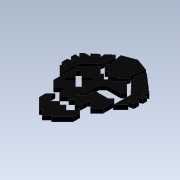
# Autodesk Inventor part: New Logo
Saved by Autodesk Inventor 2020 (Build 240168000, 168)
## iProperties
Created: 2021-10-28
Part Number: New Logo
Material: Generic
Document SubType Name: Modeling
Designer: Turing
Density: 1 g/cm^3
Appearance: Black Control Joints
Author: Turing
Autodesk Inventor part; units mm, degrees
ref_plane "YZ Plane" through (0, 0, 0) normal (1, 0, 0) x (0, 1, 0)
ref_plane "XZ Plane" through (0, 0, 0) normal (0, 1, 0) x (-1, 0, 0)
ref_plane "XY Plane" through (0, 0, 0) normal (0, 0, 1) x (1, 0, 0)
sketch "Sketch1" plane through (0, 0, 0) normal (0, 1, 0) x (-1, 0, 0)
  line L0 (0, 0) -> (-7.0711, -7.0711)
  line L1 (0, 0) -> (7.0711, -7.0711)
  line L2 (0, 0) -> (-1, 0)
  line L3 (7.0711, -7.0711) -> (17.6777, 3.5355)
  line L4 (-7.0711, -7.0711) -> (-17.6777, 3.5355)
  line L5 (0, 0) -> (0, 5)
  line L6 (0, 5) -> (7.0711, -2.0711)
  line L7 (7.0711, -2.0711) -> (17.6777, 8.5355)
  line L8 (0, 5) -> (-7.0711, -2.0711)
  line L9 (-7.0711, -2.0711) -> (-17.6777, 8.5355)
  line L10 (17.6777, 3.5355) -> (24.7487, -3.5355)
  line L11 (-17.6777, 3.5355) -> (-24.7487, -3.5355)
  line L12 (17.6777, 8.5355) -> (28.2843, -2.0711)
  line L13 (-17.6777, 8.5355) -> (-28.2843, -2.0711)
  line L14 (24.7487, -3.5355) -> (24.7487, -18.5355)
  line L15 (-24.7487, -3.5355) -> (-24.7487, -18.5355)
  line L16 (28.2843, -2.0711) -> (28.2843, -12.0711)
  line L17 (-28.2843, -2.0711) -> (-28.2843, -12.0711)
  line L18 (28.2843, -12.0711) -> (38.8909, -1.4645)
  line L19 (-28.2843, -12.0711) -> (-38.8909, -1.4645)
  line L20 (38.8909, -1.4645) -> (38.8909, 13.5355)
  line L21 (38.8909, 13.5355) -> (17.6777, 34.7487)
  line L22 (-38.8909, -1.4645) -> (-38.8909, 13.5355)
  line L23 (-38.8909, 13.5355) -> (-17.6777, 34.7487)
  line L24 (-17.6777, 34.7487) -> (17.6777, 34.7487)
  line L25 (24.7487, -18.5355) -> (28.2843, -22.0711)
  line L26 (28.2843, -22.0711) -> (42.4264, -7.9289)
  line L27 (-24.7487, -18.5355) -> (-28.2843, -22.0711)
  line L28 (-28.2843, -22.0711) -> (-42.4264, -7.9289)
  line L29 (17.6777, 34.7487) -> (14.1421, 38.2843)
  line L30 (14.1421, 38.2843) -> (10.6066, 34.7487)
  line L31 (0, 34.7487) -> (0, 45.7487)
  line L32 (10.6066, 34.7487) -> (0, 34.7487)
  line L33 (5.3033, 34.7487) -> (0, 34.7487)
  line L34 (0, 45.7487) -> (10.6066, 34.7487)
  line L35 (-17.6777, 34.7487) -> (-14.1421, 38.2843)
  line L36 (-14.1421, 38.2843) -> (-10.6066, 34.7487)
  line L37 (0, 45.7487) -> (-10.6066, 34.7487)
  line L38 (-42.4264, -7.9289) -> (-56.5685, -22.0711)
  line L39 (42.4264, -7.9289) -> (56.5685, -22.0711)
  line L40 (0, 0) -> (0, -18.5355)
  line L41 (0, -18.5355) -> (-10.6066, -29.1421)
  line L42 (-10.6066, -29.1421) -> (-10.6066, -44.1421)
  line L43 (-10.6066, -44.1421) -> (-14.1421, -47.6777)
  line L44 (-56.5685, -22.0711) -> (-56.5685, -47.6777)
  line L45 (-14.1421, -47.6777) -> (-56.5685, -47.6777)
  line L46 (-56.5685, -47.6777) -> (-49.4975, -54.7487)
  line L47 (-49.4975, -54.7487) -> (-42.4264, -47.6777)
  line L48 (-56.5685, -47.6777) -> (-52.6777, -47.6777)
  line L49 (-47.6777, -47.6777) -> (-42.4264, -47.6777)
  line L50 (-10.6066, -36.8853) -> (-5.6066, -36.8853)
  line L51 (-6.1919, -24.7274) -> (-2.6564, -28.263)
  line L52 (-5.6066, -36.8853) -> (-5.6066, -31.2132)
  line L53 (-5.6066, -31.2132) -> (-2.6564, -28.263)
  line L54 (0, -18.5355) -> (0, -25.6066)
  line L55 (0, -25.6066) -> (-2.6564, -28.263)
  line L56 (-5.6066, -36.8853) -> (-5.6066, -44.1422)
  line L57 (-5.6066, -44.1422) -> (-5.6066, -64.1422)
  line L58 (-5.6066, -64.1422) -> (-14.1421, -72.6777)
  line L59 (-14.1421, -72.6777) -> (-46.6651, -72.6777)
  line L60 (-46.6651, -72.6777) -> (-53.6117, -79.6243)
  line L61 (56.5685, -22.0711) -> (56.5685, -47.6777)
  line L62 (42.4264, -7.9289) -> (42.4264, -47.6786)
  line L63 (17.6777, 3.5355) -> (17.6777, -47.6786)
  line L64 (17.6777, -47.6786) -> (10.6066, -54.7497)
  line L65 (42.4264, -47.6786) -> (49.4975, -54.7497)
  line L66 (17.6777, -47.6786) -> (30.052, -60.053)
  line L67 (30.052, -60.053) -> (42.4264, -47.6786)
  line L68 (10.6066, -54.7497) -> (30.052, -74.1951)
  line L69 (30.052, -74.1951) -> (49.4975, -54.7497)
  line L70 (56.5685, -47.6777) -> (56.5685, -76.6674)
  line L71 (0, -25.6066) -> (0, -125.6066)
  line L72 (56.5685, -76.6674) -> (30.052, -103.1839)
  line L73 (30.052, -103.1839) -> (30.052, -74.1951)
  line L74 (30.052, -103.1839) -> (0, -103.1839)
  line L75 (0, -103.1839) -> (-30.052, -103.1839)
  line L76 (-53.6117, -79.6243) -> (-30.052, -103.1839)
  line L77 (30.052, -103.1839) -> (0, -73.1319)
  line L78 (-30.052, -103.1839) -> (0, -73.1319)
  line L79 (0, -73.1319) -> (0, -88.1319)
  line L80 (15.026, -88.1579) -> (11.4905, -91.6934)
  line L81 (11.4905, -91.6934) -> (0, -80.2029)
  line L82 (0, -80.2029) -> (-11.4905, -91.6934)
  line L83 (-11.4905, -91.6934) -> (-15.026, -88.1579)
  line L84 (0, -80.2029) -> (0, -85.2029)
  line L85 (0, -85.2029) -> (10.6066, -95.8095)
  line L86 (0, -85.2029) -> (-10.6066, -95.8095)
  line L87 (-10.6066, -95.8095) -> (-14.1421, -92.274)
  line L88 (10.6066, -95.8095) -> (14.1421, -92.274)
  line L89 (14.1421, -92.274) -> (26.87, -105.002)
  line L90 (-14.1421, -92.274) -> (-26.87, -105.002)
  line L91 (-26.87, -105.002) -> (-26.87, -110.002)
  line L92 (26.87, -105.002) -> (26.87, -110.002)
  line L93 (-26.87, -105.002) -> (-30.052, -105.002)
  line L94 (26.87, -110.002) -> (23.3345, -113.5375)
  line L95 (-26.87, -110.002) -> (-23.3345, -113.5375)
  line L96 (23.3345, -113.5375) -> (-23.3345, -113.5375)
  line L97 (0, -113.5375) -> (23.3345, -113.5375)
  line L98 (0, -113.5375) -> (-23.3345, -113.5375)
  line L99 (23.3345, -113.5375) -> (28.5439, -143.0817)
  line L100 (28.5439, -143.0817) -> (-1.5262, -154.0264)
  line L101 (-23.3345, -113.5375) -> (-28.5439, -143.0817)
  line L102 (-28.5439, -143.0817) -> (1.5262, -154.0264)
  line L103 (1.5262, -154.0264) -> (-1.5262, -154.0264)
  point P0 (0, -153.4709)
  dimension "d0" = 10
  dimension "d1" = 90
  dimension "d2" = 45
  dimension "d3" = 1
  dimension "d4" = 15
  dimension "d5" = 90
  dimension "d6" = 10
  dimension "d7" = 15
  dimension "d8" = 90
  dimension "d9" = 5
  dimension "d10" = 10
  dimension "d11" = 45
  dimension "d12" = 15
  dimension "d13" = 10
  dimension "d14" = 45
  dimension "d15" = 15
  dimension "d16" = 90
  dimension "d17" = 10
  dimension "d18" = 90
  dimension "d19" = 10
  dimension "d20" = 90
  dimension "d21" = 15
  dimension "d22" = 90
  dimension "d23" = 15
  dimension "d24" = 90
  dimension "d25" = 15
  dimension "d26" = 15
  dimension "d27" = 10
  dimension "d28" = 15
  dimension "d29" = 45
  dimension "d30" = 15
  dimension "d31" = 45
  dimension "d32" = 10
  dimension "d33" = 15
  dimension "d34" = 135
  dimension "d35" = 30
  dimension "d36" = 30
  dimension "d37" = 135
  dimension "d38" = 5
  dimension "d39" = 135
  dimension "d40" = 90
  dimension "d41" = 20
  dimension "d42" = 5
  dimension "d43" = 20
  dimension "d44" = 135
  dimension "d45" = 5
  dimension "d46" = 11
  dimension "d47" = 5
  dimension "d48" = 45
  dimension "d49" = 5
  dimension "d50" = 90
  dimension "d51" = 20
  dimension "d52" = 20
  dimension "d53" = 90
  dimension "d54" = 15
  dimension "d55" = 15
  dimension "d56" = 5
  dimension "d57" = 135
  dimension "d58" = 18.5355
  dimension "d59" = 10
  dimension "d60" = 10
  dimension "d61" = 45
  dimension "d62" = 45
  dimension "d63" = 3.8909
  constraints: 208 end point, 18 vertical, 16 point on line, 13 perpendicular, 8 horizontal, 5 collinear, 5 midpoint, 3 parallel
  measures "d0" distance of L0.start L0.end
  measures "d1" angle of L0 L1
  measures "d2" angle of L0 L2
  measures "d3" distance of L0.start L2.end
  measures "d4" distance of L1.end L3.end
  measures "d5" angle of L1 L3
  measures "d6" distance of L0.start L1.end
  measures "d7" distance of L0.end L4.end
  measures "d8" angle of L4 L0
  measures "d9" distance of L0.start L5.end
  measures "d10" distance of L5.end L6.end
  measures "d11" angle of L5 L6
  measures "d12" distance of L6.end L7.end
  measures "d13" distance of L5.end L8.end
  measures "d14" angle of L5 L8
  measures "d15" distance of L8.end L9.end
  measures "d16" angle of L6 L7
  measures "d17" distance of L3.end L10.end
  measures "d18" angle of L3 L10
  measures "d19" distance of L4.end L11.end
  measures "d20" angle of L11 L4
  measures "d21" distance of L7.end L12.end
  measures "d22" angle of L7 L12
  measures "d23" distance of L9.end L13.end
  measures "d24" angle of L13 L9
  measures "d25" distance of L10.end L14.end
  measures "d26" distance of L11.end L15.end
  measures "d27" distance of L12.end L16.end
  measures "d28" distance of L16.end L18.end
  measures "d29" angle of L16 L18
  measures "d30" distance of L17.end L19.end
  measures "d31" angle of L19 L17
  measures "d32" distance of L13.end L17.end
  measures "d33" distance of L18.end L20.end
  measures "d34" angle of L20 L21
  measures "d35" distance of L20.end L21.end
  measures "d36" distance of L22.end L23.end
  measures "d37" angle of L22 L23
  measures "d38" distance of L14.end L25.end
  measures "d39" angle of L25 L14
  measures "d40" angle of L25 L26
  measures "d41" distance of L25.end L26.end
  measures "d42" distance of L15.end L27.end
  measures "d43" distance of L27.end L28.end
  measures "d44" angle of L15 L27
  measures "d45" distance of L21.end L29.end
  measures "d46" distance of L31.start L31.end
  measures "d47" distance of L23.end L35.end
  measures "d48" angle of L24 L35
  measures "d49" distance of L35.end L36.end
  measures "d50" angle of L38 L28
  measures "d51" distance of L28.end L38.end
  measures "d52" distance of L26.end L39.end
  measures "d53" angle of L26 L39
  measures "d54" distance of L40.end L41.end
  measures "d55" distance of L41.end L42.end
  measures "d56" distance of L42.end L43.end
  measures "d57" angle of L42 L41
  measures "d58" distance of L0.start L40.end
  measures "d59" distance of L46.end L47.end
  measures "d60" distance of L44.end L46.end
  measures "d61" angle of L49 L47
  measures "d62" angle of L46 L45
  measures "d63" distance of L48.end L44.end
extrude "Extrusion1" add sketch "Sketch1" along normal blind 10 contours L40 L41 L42 L43 L45 L44 L38 L28 L27 L15 L11 L4 L0 | L8 L9 L13 L17 L19 L22 L23 L24 L21 L20 L18 L16 L12 L7 L6 | L1 L3 L63 L64 L68 L73 L77 L71 L54 L40 | L10 L14 L25 L26 L62 L67 L66 L63 | L71 L78 L76 L60 L59 L58 L57 L56 L52 L53 L55 | L77 L80 L81 L71 | L71 L82 L83 L78 | L69 L65 L62 L39 L61 L70 L72 L73 | L85 L88 L89 L74 L71 | L71 L75 L90 L87 L86 | L89 L92 L94 L96 L71 L74 | L75 L71 L96 L95 L91 L90 | L47 L46 L45 | L24 L30 L29 | L35 L36 L24 | L96 L99 L100 L102 L101 | L24 L31 L34 | L37 L31 L24
sketch "Sketch2" plane through (0, 10, 0) normal (0, 1, 0) x (1, 0, 0)
  line L0 (14.1421, 47.6777) -> (10.6066, 44.1421) projected
  line L1 (10.6066, 44.1421) -> (10.6066, 29.1421) projected
  line L2 (10.6066, 29.1421) -> (0, 18.5355) projected
  line L3 (0, 18.5355) -> (0, 25.6066) projected
  line L4 (0, 25.6066) -> (5.6066, 31.2132) projected
  line L5 (5.6066, 31.2132) -> (5.6066, 64.1422) projected
  line L6 (5.6066, 64.1422) -> (14.1421, 72.6777) projected
  line L7 (14.1421, 72.6777) -> (46.6651, 72.6777) projected
  line L8 (46.6651, 72.6777) -> (53.6117, 79.6243) projected
  line L9 (53.6117, 79.6243) -> (30.052, 103.1839) projected
  line L10 (30.052, 103.1839) -> (15.026, 88.1579) projected
  line L11 (15.026, 88.1579) -> (11.4905, 91.6934) projected
  line L12 (11.4905, 91.6934) -> (0, 80.2029) projected
  line L13 (0, 80.2029) -> (-11.4905, 91.6934) projected
  line L14 (-11.4905, 91.6934) -> (-15.026, 88.1579) projected
  line L15 (-15.026, 88.1579) -> (-30.052, 103.1839) projected
  line L16 (-30.052, 103.1839) -> (-56.5685, 76.6674) projected
  line L17 (-56.5685, 76.6674) -> (-56.5685, 22.0711) projected
  line L18 (-56.5685, 22.0711) -> (-42.4264, 7.9289) projected
  line L19 (-42.4264, 7.9289) -> (-28.2843, 22.0711) projected
  line L20 (-28.2843, 22.0711) -> (-24.7487, 18.5355) projected
  line L21 (-24.7487, 18.5355) -> (-24.7487, 3.5355) projected
  line L22 (-24.7487, 3.5355) -> (-17.6777, -3.5355) projected
  line L23 (-17.6777, -3.5355) -> (-7.0711, 7.0711) projected
  line L24 (-7.0711, 7.0711) -> (0, 0) projected
  line L25 (0, 0) -> (7.0711, 7.0711) projected
  line L26 (7.0711, 7.0711) -> (17.6777, -3.5355) projected
  line L27 (17.6777, -3.5355) -> (24.7487, 3.5355) projected
  line L28 (24.7487, 3.5355) -> (24.7487, 18.5355) projected
  line L29 (24.7487, 18.5355) -> (28.2843, 22.0711) projected
  line L30 (28.2843, 22.0711) -> (42.4264, 7.9289) projected
  line L31 (42.4264, 7.9289) -> (56.5685, 22.0711) projected
  line L32 (56.5685, 22.0711) -> (56.5685, 47.6777) projected
  line L33 (56.5685, 47.6777) -> (49.4975, 54.7487) projected
  line L34 (49.4975, 54.7487) -> (42.4264, 47.6777) projected
  line L35 (42.4264, 47.6777) -> (14.1421, 47.6777) projected
  line L36 (-30.052, 60.053) -> (-42.4264, 47.6786) projected
  line L37 (-42.4264, 47.6786) -> (-49.4975, 54.7497) projected
  line L38 (-49.4975, 54.7497) -> (-30.052, 74.1951) projected
  line L39 (-30.052, 74.1951) -> (-10.6066, 54.7497) projected
  line L40 (-10.6066, 54.7497) -> (-17.6777, 47.6786) projected
  line L41 (-17.6777, 47.6786) -> (-30.052, 60.053) projected
  line L42 (-49.4975, 40.6075) -> (-42.4264, 33.5365)
  line L43 (-30.052, 45.9108) -> (-42.4264, 33.5365)
  line L44 (-30.052, 45.9108) -> (-17.6777, 33.5365)
  line L45 (-10.6066, 40.6075) -> (-17.6777, 33.5365)
  line L46 (-10.6066, 40.6075) -> (-30.052, 60.053)
  line L47 (-30.052, 60.053) -> (-49.4975, 40.6075)
  line L48 (-10.6066, 65.3563) -> (-17.6777, 72.4273)
  line L49 (-30.052, 60.053) -> (-17.6777, 72.4273)
  line L50 (-30.052, 60.053) -> (-42.4264, 72.4273)
  line L51 (-49.4975, 65.3563) -> (-42.4264, 72.4273)
  line L52 (-49.4975, 65.3563) -> (-30.052, 45.9108)
  line L53 (-30.052, 45.9108) -> (-10.6066, 65.3563)
  point P0 (-15.9099, 60.053)
  point P1 (-22.981, 52.9819)
  point P2 (-37.1231, 67.124)
  point P3 (-22.981, 67.124)
  point P4 (-37.1231, 52.9819)
  point P5 (-44.1942, 60.053)
  constraints: 24 end point, 4 parallel, 2 perpendicular
extrude "Extrusion2" add sketch "Sketch2" against normal up to surface (10 mm away) contours L50 L38 L39 L49 | L36 L37 L38 L52 | L53 L39 L40 L41
extrude "Extrusion3" cut sketch "Sketch2" against normal up to surface (10 mm away) contours L41 L53 L52 L36 | L52 L43 L42 L47 L36 | L41 L46 L45 L44 L53 | L49 L48 L53 L39 | L38 L52 L51 L50
sketch "Sketch3" plane through (0, 10, 0) normal (0, 1, 0) x (1, 0, 0)
  line L0 (-38.8909, 1.4645) -> (-38.8909, -13.5355) projected
  line L1 (-38.8909, -13.5355) -> (-14.1421, -38.2843) projected
  line L2 (-14.1421, -38.2843) -> (-10.6066, -34.7487) projected
  line L3 (-10.6066, -34.7487) -> (0, -45.7487) projected
  line L4 (0, -45.7487) -> (10.6066, -34.7487) projected
  line L5 (10.6066, -34.7487) -> (14.1421, -38.2843) projected
  line L6 (14.1421, -38.2843) -> (38.8909, -13.5355) projected
  line L7 (38.8909, -13.5355) -> (38.8909, 1.4645) projected
  line L8 (38.8909, 1.4645) -> (28.2843, 12.0711) projected
  line L9 (28.2843, 12.0711) -> (28.2843, 2.0711) projected
  line L10 (28.2843, 2.0711) -> (17.6777, -8.5355) projected
  line L11 (17.6777, -8.5355) -> (7.0711, 2.0711) projected
  line L12 (7.0711, 2.0711) -> (0, -5) projected
  line L13 (0, -5) -> (-7.0711, 2.0711) projected
  line L14 (-7.0711, 2.0711) -> (-17.6777, -8.5355) projected
  line L15 (-17.6777, -8.5355) -> (-28.2843, 2.0711) projected
  line L16 (-28.2843, 2.0711) -> (-28.2843, 12.0711) projected
  line L17 (-28.2843, 12.0711) -> (-38.8909, 1.4645) projected
  line L18 (-38.8909, -28.3888) -> (-38.8909, -13.5355)
  line L19 (-28.2843, -2.9289) -> (-38.8909, -13.5355)
  line L20 (-28.2843, -2.9289) -> (-28.2843, -12.9289)
  line L21 (-28.2843, -12.9289) -> (-17.6777, -23.5355)
  line L22 (-7.0711, -12.9289) -> (-17.6777, -23.5355)
  line L23 (-7.0711, -12.9289) -> (0, -20)
  line L24 (7.0711, -12.9289) -> (0, -20)
  line L25 (7.0711, -12.9289) -> (17.6777, -23.5355)
  line L26 (17.6777, -23.5355) -> (28.2843, -12.9289)
  line L27 (28.2843, -2.9289) -> (28.2843, -12.9289)
  line L28 (28.2843, -2.9289) -> (38.8909, -13.5355)
  line L29 (38.8909, -13.5355) -> (38.8909, -28.5355)
  line L30 (14.1421, -53.2843) -> (38.8909, -28.5355)
  line L31 (14.1421, -53.2843) -> (10.6066, -49.7487)
  line L32 (10.6066, -49.7487) -> (0, -60.7487)
  line L33 (-10.6066, -49.7487) -> (0, -60.7487)
  line L34 (-14.0688, -53.2109) -> (-10.6066, -49.7487)
  line L35 (-38.8909, -28.3888) -> (-14.0688, -53.2109)
  line L36 (26.87, 110.002) -> (23.3345, 113.5375) projected
  line L37 (23.3345, 113.5375) -> (28.5439, 143.0817) projected
  line L38 (28.5439, 143.0817) -> (0, 153.4709) projected
  line L39 (0, 153.4709) -> (-28.5439, 143.0817) projected
  line L40 (-28.5439, 143.0817) -> (-23.3345, 113.5375) projected
  line L41 (-23.3345, 113.5375) -> (-26.87, 110.002) projected
  line L42 (-26.87, 110.002) -> (-26.87, 105.002) projected
  line L43 (-26.87, 105.002) -> (-14.1421, 92.274) projected
  line L44 (-14.1421, 92.274) -> (-10.6066, 95.8095) projected
  line L45 (-10.6066, 95.8095) -> (0, 85.2029) projected
  line L46 (0, 85.2029) -> (10.6066, 95.8095) projected
  line L47 (10.6066, 95.8095) -> (14.1421, 92.274) projected
  line L48 (14.1421, 92.274) -> (26.87, 105.002) projected
  line L49 (26.87, 105.002) -> (26.87, 110.002) projected
  line L50 (-14.1421, 97.274) -> (-26.87, 110.002)
  line L51 (-26.87, 115.002) -> (-26.87, 110.002)
  line L52 (-26.87, 115.002) -> (-23.3345, 118.5375)
  line L53 (-23.3345, 118.5375) -> (-28.5036, 147.853)
  line L54 (-28.5036, 147.853) -> (0.3344, 158.3491)
  line L55 (0.3344, 158.3491) -> (28.5439, 148.0817)
  line L56 (23.3345, 118.5375) -> (28.5439, 148.0817)
  line L57 (23.3345, 118.5375) -> (26.87, 115.002)
  line L58 (26.87, 115.002) -> (26.87, 110.002)
  line L59 (14.1421, 97.274) -> (26.87, 110.002)
  line L60 (14.1421, 97.274) -> (10.6066, 100.8095)
  line L61 (10.6066, 100.8095) -> (0, 90.2029)
  line L62 (0, 90.2029) -> (-10.6066, 100.8095)
  line L63 (-14.1421, 97.274) -> (-10.6066, 100.8095)
  point P0 (0, 0)
  point P1 (24.084, 117.788)
  point P2 (27.7155, 143.3833)
  point P3 (-27.7155, 143.3833)
  point P4 (-24.084, 117.788)
  point P5 (-26.87, 110.002)
  point P6 (26.87, 110.002)
  dimension "d128" = 15
  dimension "d133" = 5
  constraints: 64 end point, 18 parallel, 5 collinear, 5 perpendicular
  measures "d128" distance of L12.end L23.end
  measures "d133" distance of L61.end L45.end
extrude "Extrusion4" add sketch "Sketch3" against normal blind 10 contours L19 L20 L21 L22 L23 L24 L25 L26 L27 L28 L6 L5 L4 L3 L2 L1 | L1 L2 L3 L4 L5 L6 L29 L30 L31 L32 L33 L34 L35 L18 | L59 L60 L61 L62 L63 L50 L41 L40 L52 L53 L39 L38 L56 L57 L37 L36 | L36 L37 L57 L58 | L38 L39 L53 L54 L55 L56 | L51 L52 L40 L41
extrude "Extrusion5" cut sketch "Sketch3" against normal blind 10 contours L17 L16 L15 L14 L13 L12 L11 L10 L9 L8 L7 L28 L27 L26 L25 L24 L23 L22 L21 L20 L19 L0 | L49 L48 L47 L46 L45 L44 L43 L42 L50 L63 L62 L61 L60 L59 | L57 L56 L38 L37 | L53 L52 L40 L39
sketch "Sketch4" plane through (0, 10, 0) normal (0, 1, 0) x (1, 0, 0)
  line L0 (-10.6066, 65.3563) -> (-22.981, 52.9819) projected
  line L1 (-22.981, 52.9819) -> (-10.6066, 40.6075) projected
  line L2 (-10.6066, 40.6075) -> (-17.6777, 33.5365) projected
  line L3 (-17.6777, 33.5365) -> (-30.052, 45.9108) projected
  line L4 (-30.052, 45.9108) -> (-42.4264, 33.5365) projected
  line L5 (-42.4264, 33.5365) -> (-49.4975, 40.6075) projected
  line L6 (-49.4975, 40.6075) -> (-37.1231, 52.9819) projected
  line L7 (-37.1231, 52.9819) -> (-49.4975, 65.3563) projected
  line L8 (-49.4975, 65.3563) -> (-42.4264, 72.4273) projected
  line L9 (-42.4264, 72.4273) -> (-30.052, 60.053) projected
  line L10 (-30.052, 60.053) -> (-17.6777, 72.4273) projected
  line L11 (-17.6777, 72.4273) -> (-10.6066, 65.3563) projected
  line L12 (14.1421, 47.6777) -> (10.6066, 44.1421) projected
  line L13 (10.6066, 44.1421) -> (10.6066, 29.1421) projected
  line L14 (10.6066, 29.1421) -> (0, 18.5355) projected
  line L15 (0, 18.5355) -> (0, 25.6066) projected
  line L16 (0, 25.6066) -> (5.6066, 31.2132) projected
  line L17 (5.6066, 31.2132) -> (5.6066, 64.1422) projected
  line L18 (5.6066, 64.1422) -> (14.1421, 72.6777) projected
  line L19 (14.1421, 72.6777) -> (46.6651, 72.6777) projected
  line L20 (46.6651, 72.6777) -> (53.6117, 79.6243) projected
  line L21 (53.6117, 79.6243) -> (30.052, 103.1839) projected
  line L22 (30.052, 103.1839) -> (15.026, 88.1579) projected
  line L23 (15.026, 88.1579) -> (11.4905, 91.6934) projected
  line L24 (11.4905, 91.6934) -> (0, 80.2029) projected
  line L25 (0, 80.2029) -> (-11.4905, 91.6934) projected
  line L26 (-11.4905, 91.6934) -> (-15.026, 88.1579) projected
  line L27 (-15.026, 88.1579) -> (-30.052, 103.1839) projected
  line L28 (-30.052, 103.1839) -> (-56.5685, 76.6674) projected
  line L29 (-56.5685, 76.6674) -> (-56.5685, 22.0711) projected
  line L30 (-56.5685, 22.0711) -> (-42.4264, 7.9289) projected
  line L31 (-42.4264, 7.9289) -> (-28.2843, 22.0711) projected
  line L32 (-28.2843, 22.0711) -> (-24.7487, 18.5355) projected
  line L33 (-24.7487, 18.5355) -> (-24.7487, 3.5355) projected
  line L34 (-24.7487, 3.5355) -> (-17.6777, -3.5355) projected
  line L35 (-17.6777, -3.5355) -> (-7.0711, 7.0711) projected
  line L36 (-7.0711, 7.0711) -> (0, 0) projected
  line L37 (0, 0) -> (7.0711, 7.0711) projected
  line L38 (7.0711, 7.0711) -> (17.6777, -3.5355) projected
  line L39 (17.6777, -3.5355) -> (24.7487, 3.5355) projected
  line L40 (24.7487, 3.5355) -> (24.7487, 18.5355) projected
  line L41 (24.7487, 18.5355) -> (28.2843, 22.0711) projected
  line L42 (28.2843, 22.0711) -> (42.4264, 7.9289) projected
  line L43 (42.4264, 7.9289) -> (56.5685, 22.0711) projected
  line L44 (56.5685, 22.0711) -> (56.5685, 47.6777) projected
  line L45 (56.5685, 47.6777) -> (49.4975, 54.7487) projected
  line L46 (49.4975, 54.7487) -> (42.4264, 47.6777) projected
  line L47 (42.4264, 47.6777) -> (14.1421, 47.6777) projected
  line L48 (26.87, 115.002) -> (23.3345, 118.5375) projected
  line L49 (23.3345, 118.5375) -> (28.5439, 148.0817) projected
  line L50 (28.5439, 148.0817) -> (0.3344, 158.3491) projected
  line L51 (0.3344, 158.3491) -> (-28.5036, 147.853) projected
  line L52 (-28.5036, 147.853) -> (-23.3345, 118.5375) projected
  line L53 (-23.3345, 118.5375) -> (-26.87, 115.002) projected
  line L54 (-26.87, 115.002) -> (-26.87, 110.002) projected
  line L55 (-26.87, 110.002) -> (-14.1421, 97.274) projected
  line L56 (-14.1421, 97.274) -> (-10.6066, 100.8095) projected
  line L57 (-10.6066, 100.8095) -> (0, 90.2029) projected
  line L58 (0, 90.2029) -> (10.6066, 100.8095) projected
  line L59 (10.6066, 100.8095) -> (14.1421, 97.274) projected
  line L60 (14.1421, 97.274) -> (26.87, 110.002) projected
  line L61 (26.87, 110.002) -> (26.87, 115.002) projected
  line L62 (-26.87, 110.002) -> (-30.052, 110.002)
  line L63 (-30.052, 110.002) -> (-33.2341, 110.002)
  line L64 (-33.2341, 110.002) -> (-33.2341, 115.002)
  line L65 (-33.2341, 115.002) -> (-28.8497, 120.7568)
  line L66 (-33.2341, 110.002) -> (-61.5686, 81.6674)
  line L67 (-61.5686, 81.6674) -> (-61.5686, 41.6674)
  line L68 (-61.5686, 41.6674) -> (-82.7818, 62.8806)
  line L69 (-82.7818, 62.8806) -> (-82.7818, 102.8806)
  line L70 (-82.7818, 102.8806) -> (-33.0849, 144.776)
  line L71 (-33.0849, 144.776) -> (-28.8497, 120.7568)
  line L72 (-82.7818, 65.3563) -> (-72.1752, 65.3563)
  line L73 (-72.1752, 65.3563) -> (-78.7163, 58.8152)
  line L74 (-82.7818, 97.274) -> (-72.1752, 97.274)
  line L75 (-72.1752, 97.274) -> (-80.0689, 105.1677)
  line L76 (-31.824, 137.6252) -> (-35.3553, 134.0939)
  line L77 (-35.3553, 134.0939) -> (-35.3553, 142.8619)
  line L78 (-82.7818, 82.8806) -> (-72.1752, 82.8806)
  line L79 (-72.1752, 82.8806) -> (-82.7818, 79.0202)
  line L80 (-72.1752, 82.8806) -> (-82.7818, 88.1579)
  line L81 (-80.0689, 105.1677) -> (-66.3063, 116.7697)
  line L82 (-66.3063, 116.7697) -> (-61.416, 110.9687)
  line L83 (-61.416, 110.9687) -> (-73.1876, 110.9687)
  line L84 (-54.0067, 127.1385) -> (-48.6222, 121.7541)
  line L85 (-48.6222, 121.7541) -> (-48.6222, 131.6777)
  line L86 (-72.1752, 65.3563) -> (-82.7818, 67.2265)
  line L87 (0, 90.2029) -> (0.3344, 158.3491)
  line L88 (29.6159, 45.618) -> (41.8682, 33.1228)
  line L89 (41.8682, 33.1228) -> (49.0083, 40.1241)
  line L90 (49.0083, 40.1241) -> (36.756, 52.6193)
  line L91 (36.756, 52.6193) -> (49.2512, 64.8716)
  line L92 (49.2512, 64.8716) -> (42.2499, 72.0118)
  line L93 (42.2499, 72.0118) -> (29.7547, 59.7595)
  line L94 (30.178, 102.8883) -> (56.433, 76.1128)
  line L95 (27.1121, 114.737) -> (27.063, 109.7373)
  line L96 (27.063, 109.7373) -> (30.2449, 109.7061)
  line L97 (30.2449, 109.7061) -> (33.4268, 109.6748)
  line L98 (33.4268, 109.6748) -> (33.4759, 114.6746)
  line L99 (33.4759, 114.6746) -> (29.1482, 120.4722)
  line L100 (33.4268, 109.6748) -> (61.4818, 81.0636)
  line L101 (61.4818, 81.0636) -> (61.0892, 41.0655)
  line L102 (61.0892, 41.0655) -> (82.5096, 62.0695)
  line L103 (82.5096, 62.0695) -> (82.9022, 102.0675)
  line L104 (82.9022, 102.0675) -> (33.6189, 144.4486)
  line L105 (33.6189, 144.4486) -> (29.1482, 120.4722)
  line L106 (82.5339, 64.545) -> (71.9278, 64.6491)
  line L107 (71.9278, 64.6491) -> (78.4044, 58.0441)
  line L108 (82.8472, 96.4612) -> (72.2411, 96.5653)
  line L109 (72.2411, 96.5653) -> (80.2119, 104.3811)
  line L110 (32.2879, 137.3106) -> (35.7844, 133.7448)
  line L111 (35.7844, 133.7448) -> (35.8705, 142.5124)
  line L112 (82.7059, 82.0685) -> (72.0998, 82.1726)
  line L113 (72.0998, 82.1726) -> (82.668, 78.2082)
  line L114 (72.0998, 82.1726) -> (82.7577, 87.3455)
  line L115 (80.2119, 104.3811) -> (66.5639, 116.1177)
  line L116 (66.5639, 116.1177) -> (61.6168, 110.3649)
  line L117 (61.6168, 110.3649) -> (73.3879, 110.2494)
  line L118 (54.3666, 126.6067) -> (48.9295, 121.2753)
  line L119 (48.9295, 121.2753) -> (49.0269, 131.1985)
  line L120 (71.9278, 64.6491) -> (82.5523, 66.4151)
  point P0 (29.068, 147.5704)
  dimension "d134" = 3.182
  dimension "d135" = 3.182
  dimension "d136" = 40
  dimension "d137" = 45
  dimension "d138" = 30
  dimension "d139" = 40
  dimension "d140" = 65
  dimension "d141" = 0
  dimension "d142" = 82.302
  dimension "d143" = 94.869
  dimension "d144" = 18.548
  dimension "d145" = 91.9239
  dimension "d146" = 105.1908
  dimension "d147" = 118.1371
  dimension "d148" = 63.291
  dimension "d149" = 49.5964
  dimension "d150" = 17.6786
  dimension "d151" = 46.1174
  dimension "d152" = 22.5693
  dimension "d153" = 33.9645
  dimension "d154" = 65.7843
  dimension "d155" = 112.2333
  dimension "d156" = 126.1055
  constraints: 118 end point, 41 symmetric about line, 24 point on line, 7 perpendicular, 5 horizontal, 4 parallel, 3 vertical, 2 midpoint
  measures "d134" distance of L54.end L62.end
  measures "d135" distance of L62.end L63.end
  measures "d136" distance of L66.end L67.end
  measures "d137" angle of L67 L68
  measures "d138" distance of L67.end L68.end
  measures "d139" distance of L68.end L69.end
  measures "d140" distance of L69.end L70.end
  measures "d141" angle of L52 L71
  measures "d142" angle of L45 L65
  measures "d143" angle of L45 L70
  measures "d144" angle of L45 L80
  measures "d145" distance between parallel lines of L44 L77
  measures "d146" distance between parallel lines of L44 L85
  measures "d147" distance between parallel lines of L44 L67
  measures "d148" distance between parallel lines of L47 L83
  measures "d149" distance between parallel lines of L47 L74
  measures "d150" distance between parallel lines of L47 L72
  measures "d151" distance between parallel lines of L79 L51
  measures "d152" distance between parallel lines of L73 L76
  measures "d153" distance between parallel lines of L75 L84
  measures "d154" distance between parallel lines of L84 L68
  measures "d155" distance from line of L44.end L65
  measures "d156" distance from line of L44.end L76
extrude "Extrusion6" add sketch "Sketch4" against normal blind 10 contours L66 L67 L68 L73 L86 L69 L79 L80 L74 L75 L70 L83 L82 L84 L85 L77 L76 L71 L65 L64 | L98 L99 L105 L110 L111 L104 L119 L118 L116 L117 L109 L108 L103 L114 L113 L120 L107 L102 L101 L100
equation "\"d4\" = d7"
equation "\"d5\" = d1"
equation "\"d6\" = d0"
equation "\"d7\" = 1.5 * d0"
equation "\"d8\" = d1"
equation "\"d10\" = d0"
equation "\"d11\" = d2"
equation "\"d12\" = d7"
equation "\"d13\" = d0"
equation "\"d14\" = d2"
equation "\"d15\" = d7"
equation "\"d16\" = d1"
equation "\"d18\" = d1"
equation "\"d20\" = d1"
equation "\"d21\" = d7"
equation "\"d22\" = d1"
equation "\"d23\" = d7"
equation "\"d24\" = d1"
equation "\"d25\" = d7"
equation "\"d26\" = d7"
equation "\"d27\" = d0"
equation "\"d28\" = d7"
equation "\"d29\" = d2"
equation "\"d30\" = d7"
equation "\"d31\" = d2"
equation "\"d32\" = d0"
equation "\"d33\" = d7"
equation "\"d36\" = d35"
equation "\"d37\" = d34"
equation "\"d38\" = 0.5 * d0"
equation "\"d41\" = 2 * d0"
equation "\"d42\" = d38"
equation "\"d43\" = d41"
equation "\"d44\" = d39"
equation "\"d47\" = d45"
equation "\"d50\" = d1"
equation "\"d51\" = d43"
equation "\"d52\" = d43"
equation "\"d53\" = d1"
body "Solid1"
